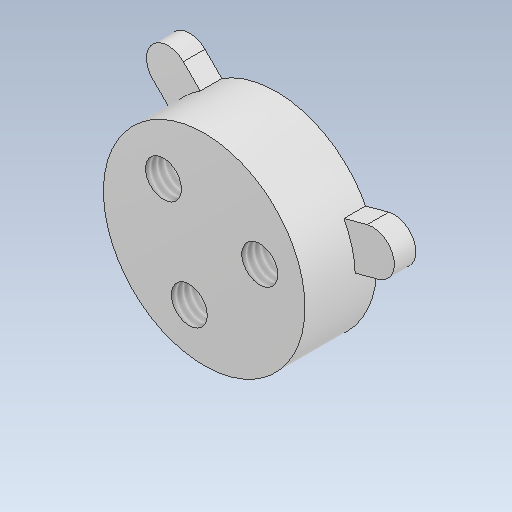
# Autodesk Inventor part: アームカムAL
Saved by Autodesk Inventor 2020.2 (Build 242310000, 310)
## iProperties
Created: 2020-03-20
Part Number: アームカムAL
Material: アルミニウム 2014-T4
Document SubType Name: Modeling
Designer: aoyam
Density: 2.8 g/cm^3
Appearance: サテン
Mass: 2.62189 g
Surface Area: 9.64862 cm^2
Volume: 0.936391 cm^3
Author: aoyam
Autodesk Inventor part; units mm, degrees
ref_plane "YZ Plane" through (0, 0, 0) normal (1, 0, 0) x (0, 1, 0)
ref_plane "XZ Plane" through (0, 0, 0) normal (0, 1, 0) x (-1, 0, 0)
ref_plane "XY Plane" through (0, 0, 0) normal (0, 0, 1) x (1, 0, 0)
sketch "スケッチ1" plane through (0, 0, 0) normal (0, 0, 1) x (1, 0, 0)
  circle A0 centre (0, 0) radius 7
  circle A1 centre (-2.8284, 2.8284) radius 1.25
  circle A2 centre (-1.0353, -3.8637) radius 1.25
  circle A3 centre (3.8637, 1.0353) radius 1.25
  circle A4 centre (0, 0) radius 10
  line L0 (3.8637, 1.0353) -> (8.2104, 2.2) construction
  line L1 (4.2519, -0.4136) -> (8.5986, 0.7511)
  line L2 (7.8221, 3.6489) -> (3.4755, 2.4842)
  arc A5 (3.4755, 2.4842) -> (4.2519, -0.4136) centre (3.8637, 1.0353) ccw
  arc A6 (8.5986, 0.7511) -> (7.8221, 3.6489) centre (8.2104, 2.2) ccw
  line L3 (3.8637, 1.0353) -> (0, 0)
  line L4 (-7.0711, 4.9497) -> (-3.8891, 1.7678)
  arc A7 (-4.9497, 7.0711) -> (-7.0711, 4.9497) centre (-6.0104, 6.0104) ccw
  line L5 (-1.7678, 3.8891) -> (-4.9497, 7.0711)
  line L6 (-0.7511, -8.5986) -> (0.4136, -4.2519)
  arc A8 (-3.6489, -7.8221) -> (-0.7511, -8.5986) centre (-2.2, -8.2104) ccw
  line L7 (-2.4842, -3.4755) -> (-3.6489, -7.8221)
  point P0 (6.037, 1.6176)
  point P1 (6.2162, 3.2185)
  point P2 (6.9926, 0.3208)
  point P3 (-3.7741, 5.8954)
  point P4 (-5.8954, 3.7741)
  point P5 (-3.2185, -6.2162)
  point P6 (-0.3208, -6.9926)
  dimension "d0" = 14
  dimension "d1" = 2.5
  dimension "d2" = 4
  dimension "d5" = 360
  dimension "d9" = 20
  dimension "d18" = 3
  dimension "d21" = 360
  constraints: 18 end point, 9 centre point, 8 point on circle, 5 tangent, 2 coincident, 1 collinear, 1 midpoint, 1 parallel, 32 other
  measures "d0" diameter of A0
  measures "d1" diameter of A1
  measures "d2" distance of A1.centre point (0, 0)
  measures "d9" diameter of A4
  measures "d18" diameter of A6
extrude "押し出し1" add sketch "スケッチ1" along normal blind 5 contours A0 L2 A5 L1 | L1 A5 L2 A0
extrude "押し出し2" add sketch "スケッチ1" along normal blind 1.5 contours A0 L2 A6 L1 | L6 A8 L7 A0 | A0 L4 A7 L5
thread "ねじ1" size "M3x0.5" class "6H" standard "ANSI Metric M Profile" full length
thread "ねじ2" size "M3x0.5" class "6H" standard "ANSI Metric M Profile" full length
thread "ねじ3" size "M3x0.5" class "6H" standard "ANSI Metric M Profile" full length
